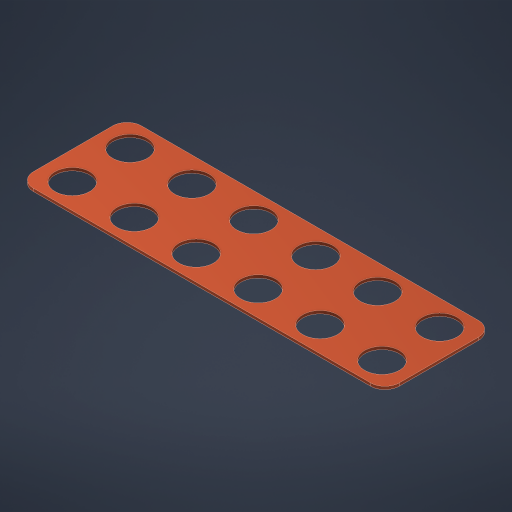
# Autodesk Inventor part: bat_contacts_v2_plate_hole
Saved by Autodesk Inventor 2024.3 (Build 283343010, 343A)
## iProperties
Created: 2025-05-07
Part Number: bat_contacts_v2_plate_hole
Material: Kupfer
Document SubType Name: Modellieren
Designer: David
Density: 8.94 g/cm^3
Appearance: Kupfer - satiniert
Sheet Metal Rule: Standard_mm
Author: David
Autodesk Inventor part; units mm, degrees
ref_plane "YZ Plane" through (0, 0, 0) normal (1, 0, 0) x (0, 1, 0)
ref_plane "XZ Plane" through (0, 0, 0) normal (0, 1, 0) x (-1, 0, 0)
ref_plane "XY Plane" through (0, 0, 0) normal (0, 0, 1) x (1, 0, 0)
sketch "Skizze1" plane through (0, 0, 0) normal (0, 0, 1) x (1, 0, 0)
  line L0 (0, 0) -> (127, 0)
  line L1 (127, 0) -> (127, 37.5)
  line L2 (127, 37.5) -> (0, 37.5)
  line L3 (0, 37.5) -> (0, 0)
  circle A0 centre (9.75, 8.75) radius 6
  circle A1 centre (31.25, 8.75) radius 6
  circle A2 centre (52.75, 8.75) radius 6
  circle A3 centre (74.25, 8.75) radius 6
  circle A4 centre (95.75, 8.75) radius 6
  circle A5 centre (117.25, 8.75) radius 6
  circle A6 centre (9.75, 28.75) radius 6
  circle A7 centre (31.25, 28.75) radius 6
  circle A8 centre (52.75, 28.75) radius 6
  circle A9 centre (74.25, 28.75) radius 6
  circle A10 centre (95.75, 28.75) radius 6
  circle A11 centre (117.25, 28.75) radius 6
  point P0 (0, 18.75)
  point P1 (63.5, 37.5)
  point P2 (42, 18.75)
  point P3 (85, 18.75)
  point P4 (63.5, 0)
  dimension "d0" = 127
  dimension "d1" = 37.5
  dimension "d17" = 43
  dimension "d18" = 21.5
  dimension "d19" = 12
  dimension "d20" = 10
  dimension "d23" = 21.5
  dimension "d26" = 20
  dimension "d29" = 10.75
  constraints: 12 centre point, 8 end point, 3 midpoint, 2 horizontal, 2 horizontal alignment, 2 parallel, 1 perpendicular, 1 vertical, 22 other
  measures "d0" distance of L1.end L2.end
  measures "d1" distance of L2.end L0.start
  measures "d17" distance of point (85, 18.75) point (42, 18.75)
  measures "d18" horizontal distance of point (63.5, 0) point (42, 18.75)
  measures "d19" diameter of A0
  measures "d20" vertical distance of point (0, 18.75) A0.centre
  measures "d23" distance of A0.centre A1.centre
  measures "d26" distance of A0.centre A6.centre
  measures "d29" horizontal distance of point (63.5, 0) A2.centre
extrude "Extrusion1" add sketch "Skizze1" along normal blind 1
fillet "Rundung1" radius 5 4 edges at (127, 37.5, 0.5) (127, 0, 0.5) (0, 37.5, 0.5) (0, 0, 0.5)
sketch "Skizze2" plane through (0, 0, 1) normal (0, 0, 1) x (1, 0, 0)
  arc A0 (0, 5) -> (5, 0) centre (5, 5) ccw projected
  line L0 (5, 0) -> (122, 0) projected
  arc A1 (122, 0) -> (127, 5) centre (122, 5) ccw projected
  line L1 (127, 5) -> (127, 32.5) projected
  arc A2 (127, 32.5) -> (122, 37.5) centre (122, 32.5) ccw projected
  line L2 (122, 37.5) -> (5, 37.5) projected
  arc A3 (5, 37.5) -> (0, 32.5) centre (5, 32.5) ccw projected
  line L3 (0, 32.5) -> (0, 5) projected
  point P0 (0, 0)
equation "\"d17\" = 2 * d9"
equation "\"d18\" = 0.5 * d17"
equation "\"d29\" = 0.5 * d23"
equation "\"Biegeradius\" = Stärke"
equation "\"BreiteBiegungsfreistellung\" = Stärke"
equation "\"TiefeBiegungsfreistellung\" = 0.5 * Stärke"
equation "\"GrößeEckenfreistellung\" = 4 * Stärke"
equation "\"MinimalRest\" = 2 * Stärke"
equation "\"Übergangsradius\" = Biegeradius"
equation "\"JacobiRadiusGröße\" = Biegeradius"
equation "\"Abstandsgröße\" = Stärke"
equation "\"Stärke\" = 0.5"
equation "\"d9\" = 21.5"
